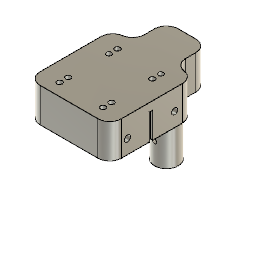
MotorTestFixture (Autodesk Fusion 360 design; units mm, degrees)
Autodesk Fusion 360 part; units mm, degrees
sketch "Sketch1" plane through (0, 0, 0) normal (0, 1, 0) x (1, 0, 0)
  line L0 (-20.5, 0) -> (20.5, 0)
  line L1 (20.5, 0) -> (20.5, -25) construction
  line L2 (20.5, -25) -> (-20.5, -25)
  line L3 (-20.5, -25) -> (-20.5, 0)
  line L4 (0, -1.75) -> (0, -22.5)
  line L5 (-30.5, -54) -> (30.5, -54)
  line L6 (30.5, -54) -> (30.5, -25) construction
  line L7 (30.5, -25) -> (-30.5, -25)
  line L8 (-30.5, -25) -> (-30.5, -54)
  line L9 (1.75, 0) -> (22.5, 0)
  line L10 (-30.5, -54) -> (-34.5, -54)
  line L11 (-34.5, -54) -> (-34.5, 0)
  line L12 (-34.5, 0) -> (-20.5, 0)
  line L13 (20.5, 0) -> (34.5, 0)
  line L14 (34.5, 0) -> (34.5, -54)
  line L15 (34.5, -54) -> (30.5, -54)
  line L16 (0, 0) -> (0, -54)
  line L17 (34.5, -25) -> (24.5, 0)
  line L18 (-34.5, -25) -> (-24.5, 0)
  point P0 (0, -25)
  dimension "d1" = 41
  dimension "d2" = 25
  dimension "d3" = 29
  dimension "d4" = 61
  dimension "d5" = 4
  dimension "d33" = 4
  dimension "d34" = 4
  constraint horizontal L0
  constraint vertical L1
  constraint horizontal L2
  constraint vertical L3
  constraint coincident L2 P0
  constraint midpoint L2 P0
  constraint coincident P0 L4
  constraint horizontal L5
  constraint vertical L6
  constraint horizontal L7
  constraint vertical L8
  constraint collinear L2 L7
  constraint midpoint P0 L7
  constraint collinear L0 L9
  constraint perpendicular L8 L10
  constraint perpendicular L10 L11
  constraint perpendicular L3 L12
  constraint perpendicular L1 L13
  constraint perpendicular L9 L14
  constraint perpendicular L14 L15
  constraint equal L12 L13
  constraint coincident L16.start origin
  constraint midpoint L5 L16.end
  constraint coincident L14 L17.start
  constraint coincident L13 L17.end
  constraint coincident L11 L18.start
  constraint coincident L12 L18.end
  constraint coincident L7 L18.start
  constraint coincident L7 L17.start
  measures "d1" distance of L1.end L3
  measures "d2" distance of L0.end L1.end
  measures "d3" distance of L5.start L7.end
  measures "d4" distance of L5.start L5.end
  measures "d5" distance of L5.start L10.end
  measures "d33" distance of L0.start L18.end
  measures "d34" distance of L0.end L17.end
extrude "Extrude1" add sketch "Sketch1" along normal mid plane 70 contours L0 L2 L3 L4 L7 L16 | L3 L7 L8 L10 L11 L12 L18 | L0 L4 L5 L9 L13 L14 L15 L16 L17 | L2 L5 L7 L8 L16 makes body 1
revolve "Revolve1" cut sketch "Sketch1" angle 360 about axis through (0, 0, 0) along (0, 0, 1) contours L0 L2 L3 L4 L7 L16 | L2 L5 L7 L8 L16 bodies 1
extrude "Extrude2" add 1 faces at (11.5, 35, 44.3333) along direction (0, 1, 0) blind 30 on bodies 1 bodies 1
sketch "Sketch2" plane through (0, 0, 54) normal (0, 0, 1) x (-1, 0, 0)
  line L0 (-34.5, -65) -> (34.5, -65)
  line L1 (34.5, -65) -> (34.5, 35)
  line L2 (34.5, 35) -> (-34.5, 35)
  line L3 (-34.5, 35) -> (-34.5, -65)
  circle A0 centre (0, 0) radius 30.5
  arc A1 (26.4138, -15.25) -> (26.4138, 15.25) centre (0, 0) ccw
  line L4 (26.4138, -15.25) -> (0, 0) construction
  line L5 (0, 0) -> (26.4138, 15.25) construction
  line L6 (30.5, 0) -> (-30.5, 0)
  arc A2 (28.1458, -16.25) -> (28.1458, 16.25) centre (0, 0) ccw
  line L7 (28.1458, -16.25) -> (26.4138, -15.25)
  line L8 (26.4138, 15.25) -> (28.1458, 16.25)
  arc A3 (-26.4138, 15.25) -> (-26.4138, -15.25) centre (0, 0) ccw
  arc A4 (-28.1458, 16.25) -> (-28.1458, -16.25) centre (0, 0) ccw
  line L9 (-28.1458, 16.25) -> (-26.4138, 15.25)
  line L10 (-26.4138, -15.25) -> (-28.1458, -16.25)
  line L11 (34.5, -1.5) -> (30.5, -1.5)
  line L12 (30.5, -1.5) -> (30.5, 1.5)
  line L13 (30.5, 1.5) -> (34.5, 1.5)
  line L14 (34.5, 1.5) -> (34.5, -1.5)
  line L15 (-34.5, 1.5) -> (-30.5, 1.5)
  line L16 (-34.5, -1.5) -> (-34.5, 1.5)
  line L17 (-30.5, -1.5) -> (-34.5, -1.5)
  line L18 (-30.5, 1.5) -> (-30.5, -1.5)
  dimension "d13" = 30
  dimension "d14" = 30
  dimension "d15" = 2
  dimension "d17" = 360
  dimension "d70" = 3
  dimension "d72" = 360
  constraint coincident A0 A1.start
  constraint coincident A0 A1.end
  constraint coincident A0.centre A1.centre
  constraint coincident L4 A2.start
  constraint coincident L5 A2.end
  constraint horizontal L11
  constraint vertical L12
  constraint horizontal L13
  constraint vertical L14
  constraint coincident L1 L11.start
  constraint midpoint L6.start L12
  measures "d13" angle of L4 L6
  measures "d14" angle of L5 L6
  measures "d15" distance of A1.start A2.start
  measures "d70" distance of L11 L13
extrude "Extrude3" cut sketch "Sketch2" against normal blind 15 contours A0 A3 A4 L10 L17 L18 | A4 L15 L17 L18 | A2 L11 L12 L13 | A0 A1 A2 L7 L11 L12 | A0 A3 A4 L9 L15 L18 | A0 A1 A2 L8 L12 L13 bodies 1
sketch "Sketch3" plane through (0, 0, 54) normal (0, 0, 1) x (-1, 0, 0)
  line L0 (-34.5, -65) -> (34.5, -65)
  line L1 (34.5, -65) -> (34.5, 35)
  line L2 (34.5, 35) -> (-34.5, 35)
  line L3 (-34.5, 35) -> (-34.5, -65)
  line L4 (26.4138, 15.25) -> (28.1458, 16.25)
  arc A0 (28.1458, -16.25) -> (28.1458, 16.25) centre (0, 0) ccw
  line L5 (28.1458, -16.25) -> (26.4138, -15.25)
  arc A1 (-26.4138, -15.25) -> (26.4138, -15.25) centre (0, 0) ccw
  line L6 (-26.4138, -15.25) -> (-28.1458, -16.25)
  arc A2 (-28.1458, 16.25) -> (-28.1458, -16.25) centre (0, 0) ccw
  line L7 (-28.1458, 16.25) -> (-26.4138, 15.25)
  arc A3 (26.4138, 15.25) -> (-26.4138, 15.25) centre (0, 0) ccw
  circle A4 centre (0, -47.5) radius 10.922
  line L8 (0, -47.5) -> (0, 0) construction
  line L9 (30.5, 0) -> (-30.5, 0)
  circle A5 centre (0, -47.5) radius 10.16
  circle A6 centre (0, -47.5) radius 13.97
  dimension "d20" = 21.844
  dimension "d21" = 17.5
  dimension "d59" = 20.32
  dimension "d62" = 27.94
  constraint coincident A4.centre L8.start
  constraint coincident A0.centre A1.centre
  constraint perpendicular L8 L9
  constraint concentric A5 A6
  measures "d20" diameter of A4
  measures "d21" distance of L0 A4.centre
  measures "d59" diameter of A5
  measures "d62" diameter of A6
extrude "Extrude4" cut sketch "Sketch3" against normal up to surface (54 mm away) contours A4 | A5 bodies 1
sketch "Sketch4" plane through (0, 65, 0) normal (0, 1, 0) x (-1, 0, 0)
  line L0 (-24.5, 0) -> (24.5, 0)
  line L1 (34.5, 54) -> (-34.5, 54)
  circle A0 centre (0, 18) radius 1.778
  line L2 (-34.5, 25) -> (-24.5, 0)
  line L3 (24.5, 0) -> (34.5, 25)
  line L4 (34.5, 25) -> (34.5, 54)
  line L5 (-34.5, 54) -> (-34.5, 25)
  circle A1 centre (0, 36) radius 1.778
  line L6 (0, 0) -> (0, 18) construction
  line L7 (0, 18) -> (0, 36) construction
  line L8 (0, 36) -> (0, 54) construction
  dimension "d24" = 3.556
  dimension "d50" = 3.556
  constraint coincident L6.start origin
  constraint coincident A0.centre L6.end
  constraint coincident A1.centre L7.end
  constraint vertical L7
  constraint midpoint L1 L8.end
  constraint equal L7 L8
  constraint equal L6 L8
  constraint collinear L7 L8
  measures "d24" diameter of A0
  measures "d50" diameter of A1
extrude "Extrude5" cut sketch "Sketch4" along normal up to surface contours A0 | A1 end surface at (-10.9084, 48.0444, 18) on bodies 1 bodies 1
sketch "Sketch5" plane through (0, 0, 54) normal (0, 0, 1) x (-1, 0, 0)
  circle A0 centre (0, -47.5) radius 10.922
  line L0 (-34.5, 35) -> (-34.5, -65)
  line L1 (-34.5, -65) -> (34.5, -65)
  line L2 (34.5, -65) -> (34.5, 35)
  line L3 (34.5, 35) -> (-34.5, 35)
  line L4 (26.4138, 15.25) -> (28.1458, 16.25)
  arc A1 (28.1458, -16.25) -> (28.1458, 16.25) centre (0, 0) ccw
  line L5 (28.1458, -16.25) -> (26.4138, -15.25)
  arc A2 (-26.4138, -15.25) -> (26.4138, -15.25) centre (0, 0) ccw
  line L6 (-26.4138, -15.25) -> (-28.1458, -16.25)
  arc A3 (-28.1458, 16.25) -> (-28.1458, -16.25) centre (0, 0) ccw
  line L7 (-28.1458, 16.25) -> (-26.4138, 15.25)
  arc A4 (26.4138, 15.25) -> (-26.4138, 15.25) centre (0, 0) ccw
  line L8 (34.5, -65) -> (17.5, -65)
  line L9 (17.5, -65) -> (17.5, -36.578)
  line L10 (17.5, -36.578) -> (34.5, -36.578)
  line L11 (34.5, -36.578) -> (34.5, -65)
  line L12 (-34.5, -36.578) -> (-17.5, -36.578)
  line L13 (-17.5, -36.578) -> (-17.5, -65)
  line L14 (-17.5, -65) -> (-34.5, -65)
  line L15 (-34.5, -65) -> (-34.5, -36.578)
  line L16 (0, -58.422) -> (0, -65) construction
  line L17 (10.922, -47.5) -> (17.5, -47.5) construction
  constraint horizontal L8
  constraint vertical L9
  constraint horizontal L10
  constraint vertical L11
  constraint coincident L1.end L2.start
  constraint horizontal L12
  constraint vertical L13
  constraint horizontal L14
  constraint vertical L15
  constraint coincident L1 L13.end
  constraint coincident L0 L12.start
  constraint collinear L10 L12
  constraint equal L10 L12
  constraint coincident A0 L16.start
  constraint coincident L1 L16.end
  constraint perpendicular L1 L16
  constraint coincident A0.centre L16
  constraint coincident A0 L17.start
  constraint coincident L9 L17.end
  constraint perpendicular L9 L17
  constraint coincident A0.centre L17
  constraint equal L16 L17
  constraint tangent A0 L10
extrude "Extrude6" cut sketch "Sketch5" against normal up to surface (54 mm away) contours L0 L1 L12 L13 L14 L15 | L1 L2 L8 L9 L10 L11 bodies 1
fillet "Fillet8" radius 10 8 edges at (-34.5, 36.578, 39.5) (-34.5, -35, 39.5) (34.5, -35, 39.5) (34.5, 36.578, 39.5) (29.5, -35, 12.5) (29.5, 36.578, 12.5) (-29.5, -35, 12.5) (-29.5, 36.578, 12.5) on bodies 1
fillet "Fillet9" radius 10 6 edges at (31.5711, 33.6491, 25.5641) (34.5, 0.789, 25) (31.5711, -32.0711, 25.5641) (-31.5711, -32.0711, 25.5641) (-34.5, 0.789, 25) (-31.5711, 33.6491, 25.5641) on bodies 1
fillet "Fillet10" radius 10 6 edges at (-17.5, 36.578, 31.7129) (-17.5, 36.4185, 4.6365) (17.5, 36.578, 31.7129) (17.5, 36.4185, 4.6365) (17.5, 65, 27) (-17.5, 65, 27) on bodies 1
extrude "Extrude7" add 1 faces at (13.719, 35.7944, 54) along direction (0, 0, 1) blind 25 separate body on bodies 1 makes body 2
extrude "Extrude9" add sketch "Sketch3" along normal up to surface (25 mm away) contours A4 | A5 bodies 2
extrude "Extrude10" add sketch "Sketch3" against normal up to surface (54 mm away) contours A5 bodies 2
extrude "Extrude11" cut sketch "Sketch3" along normal blind 5 contours A4 | A6 bodies 2
fillet "Fillet11" radius 10 1 edges at (9.4724, 43.826, 59) on bodies 2
ref_plane "WorkPlane1" through (0, 37.34, 32.6722) normal (0, -1, 0) x (1, 0, 0)
extrude "Extrude12" cut sketch "Sketch4" against normal up to surface (27.66 mm away) contours A0 | A1 bodies 2
extrude "Extrude13" cut sketch "Sketch2" along normal blind 22 contours L3 A4 L15 L16 L17 | L1 A2 L11 L13 L14 | A4 L15 L17 L18 | A2 L11 L12 L13 bodies 2
sketch "Sketch6" plane through (34.5, 0, 0) normal (1, 0, 0) x (0, 1, 0)
  line L0 (1.5, 76) -> (1.5, 54)
  line L1 (1.5, 54) -> (26.578, 54)
  line L2 (26.578, 54) -> (26.578, 79)
  line L3 (26.578, 79) -> (-25, 79)
  line L4 (-25, 79) -> (-25, 54)
  line L5 (-25, 54) -> (-1.5, 54)
  line L6 (-1.5, 54) -> (-1.5, 76)
  line L7 (-1.5, 76) -> (1.5, 76)
  circle A0 centre (-20, 66) radius 2.54
  circle A1 centre (20, 66) radius 2.54
  line L8 (20, 66) -> (-20, 66) construction
  line L9 (0, 76) -> (0, 66) construction
  dimension "d75" = 5.08
  dimension "d76" = 20
  dimension "d77" = 10
  constraint coincident A1.centre L8.start
  constraint coincident A0.centre L8.end
  constraint horizontal L8
  constraint equal A0 A1
  constraint midpoint L7 L9.start
  constraint coincident L8 L9.end
  constraint perpendicular L8 L9
  constraint midpoint L8 L9.end
  measures "d75" diameter of A0
  measures "d76" distance of A0.centre L9.end
  measures "d77" distance of L9.start L9.end
extrude "Extrude14" cut sketch "Sketch6" against normal up to surface (69 mm away) contours A0 | A1 bodies 2
sketch "Sketch9" plane through (0, 0, 79) normal (0, 0, 1) x (-1, 0, 0)
  line L0 (26.4138, 15.25) -> (28.1458, 16.25)
  arc A0 (28.1458, -16.25) -> (28.1458, 16.25) centre (0, 0) ccw
  line L1 (28.1458, -16.25) -> (26.4138, -15.25)
  arc A1 (-26.4138, -15.25) -> (26.4138, -15.25) centre (0, 0) ccw
  line L2 (-26.4138, -15.25) -> (-28.1458, -16.25)
  arc A2 (-28.1458, 16.25) -> (-28.1458, -16.25) centre (0, 0) ccw
  line L3 (-28.1458, 16.25) -> (-26.4138, 15.25)
  arc A3 (26.4138, 15.25) -> (-26.4138, 15.25) centre (0, 0) ccw
  arc A4 (7.5, -65) -> (17.5, -55) centre (7.5, -55) ccw
  line L4 (17.5, -55) -> (17.5, -46.3517)
  arc A5 (26, -36.4649) -> (17.5, -46.3517) centre (27.5, -46.3517) ccw
  arc A6 (26, -36.4649) -> (34.5, -26.578) centre (24.5, -26.578) ccw
  line L5 (34.5, -26.578) -> (34.5, 25)
  arc A7 (34.5, 25) -> (24.5, 35) centre (24.5, 25) ccw
  line L6 (24.5, 35) -> (-24.5, 35)
  arc A8 (-24.5, 35) -> (-34.5, 25) centre (-24.5, 25) ccw
  line L7 (-34.5, 25) -> (-34.5, -26.578)
  arc A9 (-34.5, -26.578) -> (-26, -36.4649) centre (-24.5, -26.578) ccw
  arc A10 (-17.5, -46.3517) -> (-26, -36.4649) centre (-27.5, -46.3517) ccw
  line L8 (-17.5, -46.3517) -> (-17.5, -55)
  arc A11 (-17.5, -55) -> (-7.5, -65) centre (-7.5, -55) ccw
  line L9 (-7.5, -65) -> (7.5, -65)
extrude "Extrude17" add sketch "Sketch9" along normal blind 4 contours L0 A0 L1 A1 L2 A2 L3 A3 | A4 L4 A5 A6 L5 A7 L6 A8 L7 A9 A10 L8 A11 L9 bodies 2
sketch "Sketch10" plane through (0, 0, 83) normal (0, 0, 1) x (1, 0, 0)
  line L0 (-24.7, 29) -> (-12, 29)
  line L1 (-12, 29) -> (-12, -29)
  line L2 (-12, -29) -> (-24.7, -29)
  line L3 (-24.7, -29) -> (-24.7, 29)
  line L4 (0, 0) -> (0, 33) construction
  line L5 (0, 0) -> (-12, 0)
  circle A0 centre (-18.35, -24.5) radius 2.25
  line L6 (-18.35, -24.5) -> (-18.35, -29) construction
  circle A1 centre (-18.35, -17.25) radius 2.25
  circle A2 centre (-18.35, 17.25) radius 2.25
  circle A3 centre (-18.35, 24.5) radius 2.25
  line L7 (-18.35, -24.5) -> (-18.35, -17.25) construction
  line L8 (-18.35, -17.25) -> (-18.35, 17.25) construction
  line L9 (-18.35, 17.25) -> (-18.35, 24.5) construction
  line L10 (-18.35, 24.5) -> (-18.35, 29) construction
  circle A4 centre (18.35, 17.25) radius 2.25
  circle A5 centre (18.35, 24.5) radius 2.25
  circle A6 centre (18.35, -17.25) radius 2.25
  circle A7 centre (18.35, -24.5) radius 2.25
  line L11 (17.5, 46.3517) -> (17.5, 55)
  arc A8 (17.5, 55) -> (7.5, 65) centre (7.5, 55) ccw
  line L12 (7.5, 65) -> (-7.5, 65)
  arc A9 (-7.5, 65) -> (-17.5, 55) centre (-7.5, 55) ccw
  line L13 (-17.5, 55) -> (-17.5, 46.3517)
  arc A10 (-26, 36.4649) -> (-17.5, 46.3517) centre (-27.5, 46.3517) ccw
  arc A11 (-26, 36.4649) -> (-34.5, 26.578) centre (-24.5, 26.578) ccw
  line L14 (-34.5, 26.578) -> (-34.5, -25)
  arc A12 (-34.5, -25) -> (-24.5, -35) centre (-24.5, -25) ccw
  line L15 (-24.5, -35) -> (24.5, -35)
  arc A13 (24.5, -35) -> (34.5, -25) centre (24.5, -25) ccw
  line L16 (34.5, -25) -> (34.5, 26.578)
  arc A14 (34.5, 26.578) -> (26, 36.4649) centre (24.5, 26.578) ccw
  arc A15 (17.5, 46.3517) -> (26, 36.4649) centre (27.5, 46.3517) ccw
  dimension "d86" = 12.7
  dimension "d87" = 58
  dimension "d88" = 12
  dimension "d89" = 4.5
  dimension "d91" = 7.25
  dimension "d94" = 34.5
  dimension "d95" = 7.25
  constraint horizontal L0
  constraint vertical L1
  constraint horizontal L2
  constraint vertical L3
  constraint coincident L4.start L5.start
  constraint vertical L4
  constraint coincident L1 L5.end
  constraint perpendicular L1 L5
  constraint midpoint L1 L5.end
  constraint coincident A0.centre L6.start
  constraint midpoint L2 L6.end
  constraint perpendicular L2 L6
  constraint equal A1 A2
  constraint equal A1 A3
  constraint equal A0 A3
  constraint coincident A1.centre L7.end
  constraint coincident A2.centre L8.end
  constraint coincident A3.centre L9.end
  constraint midpoint L0 L10.end
  constraint collinear L6 L7
  constraint collinear L7 L8
  constraint collinear L9 L10
  constraint collinear L8 L10
  constraint equal L6 L10
  constraint symmetric L4 A0 A7
  constraint symmetric L4 A1 A6
  constraint symmetric L4 A2 A4
  constraint symmetric L4 A3 A5
  measures "d86" distance of L0.start L0.end
  measures "d87" distance of L0.start L2.end
  measures "d88" distance of L4.start L5.end
  measures "d89" diameter of A0
  measures "d91" distance of A0.centre A1.centre
  measures "d94" distance of A1.centre A2.centre
  measures "d95" distance of A2.centre A3.centre
extrude "Extrude18" cut sketch "Sketch10" against normal blind 3 contours A0 | A1 | A2 | A3 | A4 | A5 | A6 | A7 bodies 2
fillet "Fillet12" radius 2 1 edges at (13.0246, 52.5518, 54) on bodies 2
hidden bodies 1
named bodies: "Motor Enclosure", "Test Fixture"
